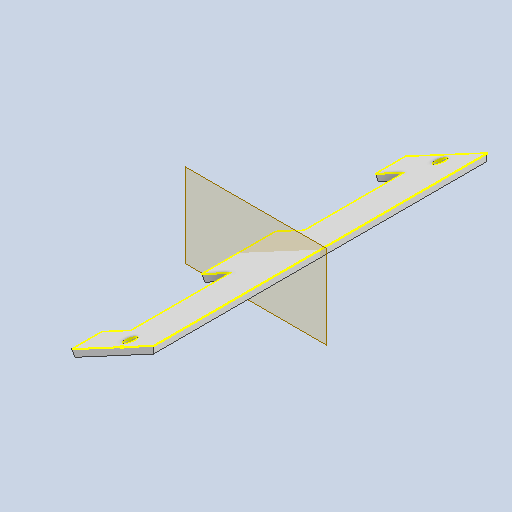
# Autodesk Inventor part: plug_2
Saved by Autodesk Inventor 2023 (Build 270158000, 158)
## iProperties
Created: 2023-07-25
Part Number: plug_2
Material: Ogólny
Document SubType Name: Modeling
Designer: Kamil
Density: 1 g/cm^3
Appearance: Domyślna
Author: Kamil
Autodesk Inventor part; units mm, degrees
ref_plane "YZ Plane" through (0, 0, 0) normal (1, 0, 0) x (0, 1, 0)
ref_plane "XZ Plane" through (0, 0, 0) normal (0, 1, 0) x (-1, 0, 0)
ref_plane "XY Plane" through (0, 0, 0) normal (0, 0, 1) x (1, 0, 0)
sketch "Szkic1" plane through (0, 0, 0) normal (0, 0, 1) x (1, 0, 0)
  line L0 (0, 0) -> (0, -66.5) projected
  line L1 (0, -66.5) -> (2, -66.5) projected
  line L2 (2, 0) -> (2, -66.5) projected
  line L3 (0, 0) -> (2, 0) projected
  circle A0 centre (7, 15.8) radius 1.5 projected
  circle A1 centre (7, 15.8) radius 15.02 projected
  line L4 (7, 30.82) -> (7, 14.3)
  line L5 (7, -69.18) -> (-7.0129, -69.18)
  line L6 (37, -46.3508) -> (4.3309, -63.8229) projected
  line L7 (37, -48.6189) -> (3.5105, -66.5297) projected
  line L8 (37, -48.6189) -> (37, -46.3508)
  line L9 (37, -48.6189) -> (-1.4451, -69.18)
  line L10 (37, -46.3508) -> (-1.4451, -66.9119)
  line L11 (-1.4451, -66.9119) -> (-1.4451, -69.18)
  dimension "d0" = 100
  constraints: 12 end point, 3 point on line, 2 vertical, 2 vertical alignment, 1 parallel, 1 perpendicular, 2 other
  measures "d0" distance of L4.start L5.start
extrude "Wyciągnięcie proste1" add sketch "Szkic1" against normal blind 100 contours L10 L2 L1 L0 | L0 L1 L2 L10 L6 L8 L7 L9 L11
sketch "Szkic5" plane through (-1.4451, -69.18, -100) normal (0.4716076, -0.8818085, 0) x (0.8818085, 0.4716076, 0)
  line L0 (17.9345, 9.0111) -> (17.7164, 38.6148) projected
  line L1 (17.7164, 38.6148) -> (26.2335, 38.9662) projected
  line L2 (26.4517, 9.3625) -> (17.9345, 9.0111) projected
  line L3 (26.2335, 38.9662) -> (17.9345, 38.9662)
  line L4 (17.9345, 38.9662) -> (17.9345, 9.0111)
  line L5 (17.9345, 9.0111) -> (26.2335, 9.0111)
  line L6 (26.2335, 9.0111) -> (26.2335, 38.9662)
  line L7 (17.4345, 39.4662) -> (26.7335, 39.4662)
  line L8 (26.7335, 39.4662) -> (26.7335, 8.5111)
  line L9 (26.7335, 8.5111) -> (17.4345, 8.5111)
  line L10 (17.4345, 8.5111) -> (17.4345, 39.4662)
  line L11 (17.4345, 39.4662) -> (16.9345, 39.4662)
  line L12 (16.9345, 39.4662) -> (16.9345, 8.5111)
  line L13 (16.9345, 8.5111) -> (17.4345, 8.5111)
  line L14 (17.4345, 8.5111) -> (17.4345, 39.4662)
  line L15 (26.7335, 38.9662) -> (16.9345, 38.9662)
  line L16 (16.9345, 38.9662) -> (16.9345, 9.0111)
  line L17 (16.9345, 9.0111) -> (26.7335, 9.0111)
  line L18 (26.7335, 9.0111) -> (26.7335, 38.9662)
  point P0 (33.9001, 100)
  point P1 (17.9345, 9.0111)
  point P2 (26.7335, 9.0111)
  point P3 (17.9345, 38.9662)
  dimension "d7" = 0.5
  dimension "d8" = 0.5
  constraints: 32 end point, 8 parallel, 4 perpendicular, 3 horizontal, 2 point on line, 3 other
  measures "d7" distance between parallel lines of L3 L7
  measures "d8" distance of L13.end L12.end
extrude "Wyciągnięcie proste4" cut sketch "Szkic5" against normal through all contours L17 L10 L15 L4 L1 L0 | L4 L1 L6 L2 | L0 L1 L4 | L2 L6 L5 | L6 L15 L8 L17 | L4 L3 L1 | L17 L12 L15 L10
ref_plane "Płaszczyzna konstrukcyjna1" through (0, 0, -50) normal (0, 0, 1) x (1, 0, 0)
mirror "Odbij1" about plane through (0, 0, -50) normal (0, 0, 1) of "Wyciągnięcie proste4"
sketch "Szkic6" plane through (-1.4451, -69.18, -100) normal (0.4716076, -0.8818085, 0) x (0.8818085, 0.4716076, 0)
  line L0 (0, 100) -> (1.0696, 100) projected
  line L1 (0, 100) -> (0, 0) projected
  line L2 (1.0696, 0) -> (0, 0) projected
  line L3 (1.0696, 0) -> (44.6676, 0) projected
  line L4 (0, 100) -> (16.9345, 100)
  line L5 (16.9345, 100) -> (16.9345, 0)
  line L6 (16.9345, 0) -> (0, 0)
  line L7 (0, 0) -> (0, 100)
  line L8 (0, 0) -> (1.0696, 0) projected
  line L9 (0, 0) -> (-9.525, 0)
  line L10 (-9.525, 0) -> (-9.525, 100)
  line L11 (-9.525, 100) -> (0, 100)
  line L12 (0, 100) -> (0, 0)
  line L13 (1.0696, 0) -> (1.0696, 100) projected
  point P0 (33.9001, 100)
  point P1 (43.598, 0)
  point P2 (16.9345, 0)
  point P3 (0, 100)
  point P4 (16.9345, 61.0338)
  point P5 (16.9345, 90.9889)
  point P6 (16.9345, 9.0111)
  point P7 (16.9345, 38.9662)
  constraints: 16 end point, 4 parallel, 2 horizontal, 2 perpendicular, 2 point on line
extrude "Wyciągnięcie proste5" cut sketch "Szkic6" against normal through all
sketch "Szkic7" plane through (37, -48.6189, -100) normal (0.4716076, -0.8818085, 0) x (0.8818085, 0.4716076, 0)
  line L0 (-26.6634, 90.9889) -> (-16.8645, 90.9889) projected
  line L1 (-16.8645, 90.9889) -> (-16.8645, 61.0338) projected
  line L2 (-16.8645, 61.0338) -> (-26.6634, 61.0338) projected
  line L3 (-26.6634, 38.9662) -> (-16.8645, 38.9662) projected
  line L4 (-16.8645, 38.9662) -> (-16.8645, 9.0111) projected
  line L5 (-16.8645, 9.0111) -> (-26.6634, 9.0111) projected
  line L6 (0, 0) -> (-26.6634, 0) projected
  line L7 (0, 100) -> (0, 0) projected
  line L8 (-26.6634, 100) -> (0, 100) projected
  line L9 (-26.6634, 90.9889) -> (-26.6634, 100) projected
  line L10 (0, 100) -> (-26.6634, 100)
  line L11 (-26.6634, 100) -> (-26.6634, 92.9)
  line L12 (-26.6634, 92.9) -> (0, 92.9)
  line L13 (0, 92.9) -> (0, 100)
  line L14 (-16.8645, 90.9889) -> (-16.8645, 100)
  line L15 (1.0696, 100) -> (-42.5283, 100) projected
  circle A0 centre (-11, 96.45) radius 1.75
  line L16 (-52.6978, 50) -> (11.0012, 50) projected
  circle A1 centre (-11, 3.55) radius 1.75
  line L17 (-26.6634, 100) -> (-26.6634, 90.9889) projected
  line L18 (-26.6634, 61.0338) -> (-26.6634, 38.9662) projected
  line L19 (-26.6634, 9.0111) -> (-26.6634, 0) projected
  point P0 (-9.6979, 100)
  point P1 (0, 96.45)
  dimension "d13" = 7.1
  dimension "d15" = 11
  dimension "d16" = 3.55
  dimension "d17" = 3.5
  constraints: 10 end point, 2 centre point, 2 parallel, 2 perpendicular, 2 point on line, 1 horizontal, 1 midpoint, 1 symmetric about line, 1 other
  measures "d13" distance of L11.end L10.end
  measures "d15" distance of point (0, 96.45) A0.centre
  measures "d16" distance from line of A0.centre L10
  measures "d17" diameter of A0
extrude "Wyciągnięcie proste6" cut sketch "Szkic7" against normal through all contours A0 | A1
sketch "Szkic8" plane through (37, -46.3508, 0) normal (-0.4716076, 0.8818085, 0) x (0.8818085, 0.4716076, 0)
  circle A0 centre (-12.0696, 96.45) radius 1.75 projected
  circle A1 centre (-12.0696, 3.55) radius 1.75 projected
  line L0 (-27.7331, 9.0111) -> (-27.7331, 0) projected
  line L1 (0, 0) -> (-27.7331, 0) projected
  line L2 (0, 0) -> (0, 100) projected
  line L3 (-27.7331, 100) -> (0, 100) projected
  line L4 (-27.7331, 100) -> (-27.7331, 90.9889) projected
  line L5 (-27.7331, 90.9889) -> (-17.9341, 90.9889) projected
  line L6 (-17.9341, 90.9889) -> (-17.9341, 61.0338) projected
  line L7 (-17.9341, 61.0338) -> (-27.7331, 61.0338) projected
  line L8 (-27.7331, 61.0338) -> (-27.7331, 38.9662) projected
  line L9 (-27.7331, 38.9662) -> (-17.9341, 38.9662) projected
  line L10 (-17.9341, 38.9662) -> (-17.9341, 9.0111) projected
  line L11 (-17.9341, 9.0111) -> (-27.7331, 9.0111) projected
  point P0 (-10.7675, 0)
